Autodesk Fusion 360 part; units mm, degrees
note: some values were not read from the file. Set by a fixed rule: which face or edge a step refers to.
(part 12 of 12)
sketch "Sketch1 (2)" plane through (0, 0, 0) normal (0, 0, 1) x (1, 0, 0) in component "Component"
  spline S0 degree 5 poles (12.8573, -1.2306) (12.8574, -1.2306) (12.8577, -1.2307) (12.8582, -1.2307) (12.8589, -1.2308) (12.8601, -1.2308) (12.8614, -1.2309) (12.8628, -1.231) (12.8645, -1.2311) (12.8663, -1.2312) (12.8683, -1.2313) (12.8704, -1.2315) (12.8727, -1.2316) (12.8752, -1.2317) (12.8778, -1.2318) (12.8806, -1.2319) (12.8835, -1.232) (12.8866, -1.2321) (12.8898, -1.2321) (12.8931, -1.2322) (12.8966, -1.2323) (12.9003, -1.2323) (12.904, -1.2324) (12.9079, -1.2324) (12.912, -1.2324) (12.9161, -1.2324) (12.9204, -1.2324) (12.9248, -1.2324) (12.9294, -1.2323) (12.9341, -1.2323) (12.9389, -1.2322) (12.9438, -1.2321) (12.9488, -1.232) (12.954, -1.2318) (12.9592, -1.2317) (12.9646, -1.2315) (12.9701, -1.2313) (12.9757, -1.2311) (12.9814, -1.2309) (12.9873, -1.2306) (12.9932, -1.2303) (12.9992, -1.23) (13.0054, -1.2296) (13.0117, -1.2293) (13.018, -1.2289) (13.0245, -1.2285) (13.031, -1.228) (13.0377, -1.2276) (13.0444, -1.2271) (13.0513, -1.2265) (13.0583, -1.226) (13.0653, -1.2254) (13.0724, -1.2248) (13.0797, -1.2241) (13.087, -1.2234) (13.0944, -1.2227) (13.1019, -1.222) (13.1095, -1.2212) (13.1172, -1.2204) (13.125, -1.2196) (13.1329, -1.2187) (13.1408, -1.2178) (13.1488, -1.2169) (13.157, -1.2159) (13.1652, -1.2149) (13.1734, -1.2138) (13.1818, -1.2128) (13.1903, -1.2117) (13.1988, -1.2105) (13.2074, -1.2093) (13.2161, -1.2081) (13.2248, -1.2068) (13.2337, -1.2056) (13.2426, -1.2042) (13.2516, -1.2029) (13.2606, -1.2014) (13.2698, -1.2) (13.279, -1.1985) (13.2883, -1.197) (13.2976, -1.1954) (13.307, -1.1938) (13.3165, -1.1922) (13.3261, -1.1905) (13.3358, -1.1888) (13.3455, -1.187) (13.3552, -1.1852) (13.3651, -1.1834) (13.375, -1.1815) (13.385, -1.1796) (13.395, -1.1776) (13.4051, -1.1756) (13.4153, -1.1736) (13.4255, -1.1715) (13.4358, -1.1694) (13.4462, -1.1672) (13.4566, -1.165) (13.4671, -1.1627) (13.4776, -1.1604) (13.4882, -1.1581) (13.4989, -1.1557) (13.5096, -1.1533) (13.5204, -1.1508) (13.5312, -1.1483) (13.5421, -1.1457) (13.5531, -1.1431) (13.5641, -1.1404) (13.5752, -1.1377) (13.5863, -1.135) (13.5975, -1.1322) (13.6087, -1.1294) (13.62, -1.1265) (13.6313, -1.1236) (13.6427, -1.1206) (13.6542, -1.1176) (13.6657, -1.1146) (13.6772, -1.1115) (13.6888, -1.1083) (13.7005, -1.1051) (13.7122, -1.1019) (13.7239, -1.0986) (13.7357, -1.0953) (13.7476, -1.0919) (13.7595, -1.0885) (13.7714, -1.085) (13.7834, -1.0815) (13.7955, -1.0779) (13.8076, -1.0743) (13.8197, -1.0706) (13.8319, -1.0669) (13.8441, -1.0631) (13.8564, -1.0593) (13.8687, -1.0555) (13.8811, -1.0516) (13.8935, -1.0476) (13.9059, -1.0436) (13.9184, -1.0396) (13.931, -1.0355) (13.9435, -1.0314) (13.9562, -1.0272) (13.9688, -1.0229) (13.9815, -1.0186) (13.9943, -1.0143) (14.0071, -1.0099) (14.0199, -1.0055) (14.0328, -1.001) (14.0457, -0.9965) (14.0586, -0.9919) (14.0716, -0.9873) (14.0846, -0.9826) (14.0977, -0.9778) (14.1108, -0.9731) (14.1239, -0.9682) (14.1371, -0.9634) (14.1503, -0.9584) (14.1635, -0.9534) (14.1768, -0.9484) (14.1901, -0.9433) (14.2035, -0.9382) (14.2168, -0.933) (14.2303, -0.9278) (14.2437, -0.9225) (14.2572, -0.9172) (14.2707, -0.9118) (14.2843, -0.9064) (14.2979, -0.9009) (14.3115, -0.8954) (14.3251, -0.8898) (14.3388, -0.8842) (14.3525, -0.8785) (14.3663, -0.8727) (14.38, -0.8669) (14.3938, -0.8611) (14.4077, -0.8552) (14.4216, -0.8493) (14.4354, -0.8433) (14.4494, -0.8373) (14.4633, -0.8312) (14.4773, -0.825) (14.4913, -0.8188) (14.5054, -0.8126) (14.5194, -0.8063) (14.5335, -0.7999) (14.5476, -0.7935) (14.5618, -0.7871) (14.576, -0.7806) (14.5902, -0.774) (14.6044, -0.7674) (14.6186, -0.7608) (14.6329, -0.754) (14.6472, -0.7473) (14.6615, -0.7405) (14.6759, -0.7336) (14.6903, -0.7267) (14.7047, -0.7197) (14.7191, -0.7127) (14.7336, -0.7056) (14.748, -0.6985) (14.7625, -0.6913) (14.777, -0.6841) (14.7916, -0.6768) (14.8061, -0.6695) (14.8207, -0.6621) (14.8353, -0.6547) (14.8499, -0.6472) (14.8646, -0.6396) (14.8793, -0.632) (14.894, -0.6244) (14.9087, -0.6167) (14.9234, -0.609) (14.9381, -0.6011) (14.9529, -0.5933) (14.9677, -0.5854) (14.9825, -0.5774) (14.9973, -0.5694) (15.0122, -0.5614) (15.027, -0.5532) (15.0419, -0.5451) (15.0568, -0.5368) (15.0717, -0.5286) (15.0867, -0.5202) (15.1016, -0.5119) (15.1166, -0.5034) (15.1316, -0.495) (15.1466, -0.4864) (15.1616, -0.4778) (15.1766, -0.4692) (15.1916, -0.4605) (15.2067, -0.4518) (15.2218, -0.443) (15.2369, -0.4341) (15.252, -0.4252) (15.2671, -0.4162) (15.2822, -0.4072) (15.2974, -0.3982) (15.3125, -0.3891) (15.3277, -0.3799) (15.3429, -0.3707) (15.3581, -0.3614) (15.3733, -0.3521) (15.3885, -0.3427) (15.4038, -0.3333) (15.416, -0.3257) (15.4251, -0.32) (15.4312, -0.3162) (15.4343, -0.3143) knots 0 0 0 0 0 0 0.00416667 0.00833333 0.0125 0.01666667 0.02083333 0.025 0.02916667 0.03333333 0.0375 0.04166667 0.04583333 0.05 0.05416667 0.05833333 0.0625 0.06666667 0.07083333 0.075 0.07916667 0.08333333 0.0875 0.09166667 0.09583333 0.1 0.10416667 0.10833333 0.1125 0.11666667 0.12083333 0.125 0.12916667 0.13333333 0.1375 0.14166667 0.14583333 0.15 0.15416667 0.15833333 0.1625 0.16666667 0.17083333 0.175 0.17916667 0.18333333 0.1875 0.19166667 0.19583333 0.2 0.20416667 0.20833333 0.2125 0.21666667 0.22083333 0.225 0.22916667 0.23333333 0.2375 0.24166667 0.24583333 0.25 0.25416667 0.25833333 0.2625 0.26666667 0.27083333 0.275 0.27916667 0.28333333 0.2875 0.29166667 0.29583333 0.3 0.30416667 0.30833333 0.3125 0.31666667 0.32083333 0.325 0.32916667 0.33333333 0.3375 0.34166667 0.34583333 0.35 0.35416667 0.35833333 0.3625 0.36666667 0.37083333 0.375 0.37916667 0.38333333 0.3875 0.39166667 0.39583333 0.4 0.40416667 0.40833333 0.4125 0.41666667 0.42083333 0.425 0.42916667 0.43333333 0.4375 0.44166667 0.44583333 0.45 0.45416667 0.45833333 0.4625 0.46666667 0.47083333 0.475 0.47916667 0.48333333 0.4875 0.49166667 0.49583333 0.5 0.50416667 0.50833333 0.5125 0.51666667 0.52083333 0.525 0.52916667 0.53333333 0.5375 0.54166667 0.54583333 0.55 0.55416667 0.55833333 0.5625 0.56666667 0.57083333 0.575 0.57916667 0.58333333 0.5875 0.59166667 0.59583333 0.6 0.60416667 0.60833333 0.6125 0.61666667 0.62083333 0.625 0.62916667 0.63333333 0.6375 0.64166667 0.64583333 0.65 0.65416667 0.65833333 0.6625 0.66666667 0.67083333 0.675 0.67916667 0.68333333 0.6875 0.69166667 0.69583333 0.7 0.70416667 0.70833333 0.7125 0.71666667 0.72083333 0.725 0.72916667 0.73333333 0.7375 0.74166667 0.74583333 0.75 0.75416667 0.75833333 0.7625 0.76666667 0.77083333 0.775 0.77916667 0.78333333 0.7875 0.79166667 0.79583333 0.8 0.80416667 0.80833333 0.8125 0.81666667 0.82083333 0.825 0.82916667 0.83333333 0.8375 0.84166667 0.84583333 0.85 0.85416667 0.85833333 0.8625 0.86666667 0.87083333 0.875 0.87916667 0.88333333 0.8875 0.89166667 0.89583333 0.9 0.90416667 0.90833333 0.9125 0.91666667 0.92083333 0.925 0.92916667 0.93333333 0.9375 0.94166667 0.94583333 0.95 0.95416667 0.95833333 0.9625 0.96666667 0.97083333 0.975 0.97916667 0.98333333 0.9875 0.99166667 0.99583333 1 1 1 1 1 1
  spline S1 degree 5 poles (12.8573, 1.2306) (12.8574, 1.2306) (12.8577, 1.2307) (12.8582, 1.2307) (12.8589, 1.2308) (12.8601, 1.2308) (12.8614, 1.2309) (12.8628, 1.231) (12.8645, 1.2311) (12.8663, 1.2312) (12.8683, 1.2313) (12.8704, 1.2315) (12.8727, 1.2316) (12.8752, 1.2317) (12.8778, 1.2318) (12.8806, 1.2319) (12.8835, 1.232) (12.8866, 1.2321) (12.8898, 1.2321) (12.8931, 1.2322) (12.8966, 1.2323) (12.9003, 1.2323) (12.904, 1.2324) (12.9079, 1.2324) (12.912, 1.2324) (12.9161, 1.2324) (12.9204, 1.2324) (12.9248, 1.2324) (12.9294, 1.2323) (12.9341, 1.2323) (12.9389, 1.2322) (12.9438, 1.2321) (12.9488, 1.232) (12.954, 1.2318) (12.9592, 1.2317) (12.9646, 1.2315) (12.9701, 1.2313) (12.9757, 1.2311) (12.9814, 1.2309) (12.9873, 1.2306) (12.9932, 1.2303) (12.9992, 1.23) (13.0054, 1.2296) (13.0117, 1.2293) (13.018, 1.2289) (13.0245, 1.2285) (13.031, 1.228) (13.0377, 1.2276) (13.0444, 1.2271) (13.0513, 1.2265) (13.0583, 1.226) (13.0653, 1.2254) (13.0724, 1.2248) (13.0797, 1.2241) (13.087, 1.2234) (13.0944, 1.2227) (13.1019, 1.222) (13.1095, 1.2212) (13.1172, 1.2204) (13.125, 1.2196) (13.1329, 1.2187) (13.1408, 1.2178) (13.1488, 1.2169) (13.157, 1.2159) (13.1652, 1.2149) (13.1734, 1.2138) (13.1818, 1.2128) (13.1903, 1.2117) (13.1988, 1.2105) (13.2074, 1.2093) (13.2161, 1.2081) (13.2248, 1.2068) (13.2337, 1.2056) (13.2426, 1.2042) (13.2516, 1.2029) (13.2606, 1.2014) (13.2698, 1.2) (13.279, 1.1985) (13.2883, 1.197) (13.2976, 1.1954) (13.307, 1.1938) (13.3165, 1.1922) (13.3261, 1.1905) (13.3358, 1.1888) (13.3455, 1.187) (13.3552, 1.1852) (13.3651, 1.1834) (13.375, 1.1815) (13.385, 1.1796) (13.395, 1.1776) (13.4051, 1.1756) (13.4153, 1.1736) (13.4255, 1.1715) (13.4358, 1.1694) (13.4462, 1.1672) (13.4566, 1.165) (13.4671, 1.1627) (13.4776, 1.1604) (13.4882, 1.1581) (13.4989, 1.1557) (13.5096, 1.1533) (13.5204, 1.1508) (13.5312, 1.1483) (13.5421, 1.1457) (13.5531, 1.1431) (13.5641, 1.1404) (13.5752, 1.1377) (13.5863, 1.135) (13.5975, 1.1322) (13.6087, 1.1294) (13.62, 1.1265) (13.6313, 1.1236) (13.6427, 1.1206) (13.6542, 1.1176) (13.6657, 1.1146) (13.6772, 1.1115) (13.6888, 1.1083) (13.7005, 1.1051) (13.7122, 1.1019) (13.7239, 1.0986) (13.7357, 1.0953) (13.7476, 1.0919) (13.7595, 1.0885) (13.7714, 1.085) (13.7834, 1.0815) (13.7955, 1.0779) (13.8076, 1.0743) (13.8197, 1.0706) (13.8319, 1.0669) (13.8441, 1.0631) (13.8564, 1.0593) (13.8687, 1.0555) (13.8811, 1.0516) (13.8935, 1.0476) (13.9059, 1.0436) (13.9184, 1.0396) (13.931, 1.0355) (13.9435, 1.0314) (13.9562, 1.0272) (13.9688, 1.0229) (13.9815, 1.0186) (13.9943, 1.0143) (14.0071, 1.0099) (14.0199, 1.0055) (14.0328, 1.001) (14.0457, 0.9965) (14.0586, 0.9919) (14.0716, 0.9873) (14.0846, 0.9826) (14.0977, 0.9778) (14.1108, 0.9731) (14.1239, 0.9682) (14.1371, 0.9634) (14.1503, 0.9584) (14.1635, 0.9534) (14.1768, 0.9484) (14.1901, 0.9433) (14.2035, 0.9382) (14.2168, 0.933) (14.2303, 0.9278) (14.2437, 0.9225) (14.2572, 0.9172) (14.2707, 0.9118) (14.2843, 0.9064) (14.2979, 0.9009) (14.3115, 0.8954) (14.3251, 0.8898) (14.3388, 0.8842) (14.3525, 0.8785) (14.3663, 0.8727) (14.38, 0.8669) (14.3938, 0.8611) (14.4077, 0.8552) (14.4216, 0.8493) (14.4354, 0.8433) (14.4494, 0.8373) (14.4633, 0.8312) (14.4773, 0.825) (14.4913, 0.8188) (14.5054, 0.8126) (14.5194, 0.8063) (14.5335, 0.7999) (14.5476, 0.7935) (14.5618, 0.7871) (14.576, 0.7806) (14.5902, 0.774) (14.6044, 0.7674) (14.6186, 0.7608) (14.6329, 0.754) (14.6472, 0.7473) (14.6615, 0.7405) (14.6759, 0.7336) (14.6903, 0.7267) (14.7047, 0.7197) (14.7191, 0.7127) (14.7336, 0.7056) (14.748, 0.6985) (14.7625, 0.6913) (14.777, 0.6841) (14.7916, 0.6768) (14.8061, 0.6695) (14.8207, 0.6621) (14.8353, 0.6547) (14.8499, 0.6472) (14.8646, 0.6396) (14.8793, 0.632) (14.894, 0.6244) (14.9087, 0.6167) (14.9234, 0.609) (14.9381, 0.6011) (14.9529, 0.5933) (14.9677, 0.5854) (14.9825, 0.5774) (14.9973, 0.5694) (15.0122, 0.5614) (15.027, 0.5532) (15.0419, 0.5451) (15.0568, 0.5368) (15.0717, 0.5286) (15.0867, 0.5202) (15.1016, 0.5119) (15.1166, 0.5034) (15.1316, 0.495) (15.1466, 0.4864) (15.1616, 0.4778) (15.1766, 0.4692) (15.1916, 0.4605) (15.2067, 0.4518) (15.2218, 0.443) (15.2369, 0.4341) (15.252, 0.4252) (15.2671, 0.4162) (15.2822, 0.4072) (15.2974, 0.3982) (15.3125, 0.3891) (15.3277, 0.3799) (15.3429, 0.3707) (15.3581, 0.3614) (15.3733, 0.3521) (15.3885, 0.3427) (15.4038, 0.3333) (15.416, 0.3257) (15.4251, 0.32) (15.4312, 0.3162) (15.4343, 0.3143) knots 0 0 0 0 0 0 0.00416667 0.00833333 0.0125 0.01666667 0.02083333 0.025 0.02916667 0.03333333 0.0375 0.04166667 0.04583333 0.05 0.05416667 0.05833333 0.0625 0.06666667 0.07083333 0.075 0.07916667 0.08333333 0.0875 0.09166667 0.09583333 0.1 0.10416667 0.10833333 0.1125 0.11666667 0.12083333 0.125 0.12916667 0.13333333 0.1375 0.14166667 0.14583333 0.15 0.15416667 0.15833333 0.1625 0.16666667 0.17083333 0.175 0.17916667 0.18333333 0.1875 0.19166667 0.19583333 0.2 0.20416667 0.20833333 0.2125 0.21666667 0.22083333 0.225 0.22916667 0.23333333 0.2375 0.24166667 0.24583333 0.25 0.25416667 0.25833333 0.2625 0.26666667 0.27083333 0.275 0.27916667 0.28333333 0.2875 0.29166667 0.29583333 0.3 0.30416667 0.30833333 0.3125 0.31666667 0.32083333 0.325 0.32916667 0.33333333 0.3375 0.34166667 0.34583333 0.35 0.35416667 0.35833333 0.3625 0.36666667 0.37083333 0.375 0.37916667 0.38333333 0.3875 0.39166667 0.39583333 0.4 0.40416667 0.40833333 0.4125 0.41666667 0.42083333 0.425 0.42916667 0.43333333 0.4375 0.44166667 0.44583333 0.45 0.45416667 0.45833333 0.4625 0.46666667 0.47083333 0.475 0.47916667 0.48333333 0.4875 0.49166667 0.49583333 0.5 0.50416667 0.50833333 0.5125 0.51666667 0.52083333 0.525 0.52916667 0.53333333 0.5375 0.54166667 0.54583333 0.55 0.55416667 0.55833333 0.5625 0.56666667 0.57083333 0.575 0.57916667 0.58333333 0.5875 0.59166667 0.59583333 0.6 0.60416667 0.60833333 0.6125 0.61666667 0.62083333 0.625 0.62916667 0.63333333 0.6375 0.64166667 0.64583333 0.65 0.65416667 0.65833333 0.6625 0.66666667 0.67083333 0.675 0.67916667 0.68333333 0.6875 0.69166667 0.69583333 0.7 0.70416667 0.70833333 0.7125 0.71666667 0.72083333 0.725 0.72916667 0.73333333 0.7375 0.74166667 0.74583333 0.75 0.75416667 0.75833333 0.7625 0.76666667 0.77083333 0.775 0.77916667 0.78333333 0.7875 0.79166667 0.79583333 0.8 0.80416667 0.80833333 0.8125 0.81666667 0.82083333 0.825 0.82916667 0.83333333 0.8375 0.84166667 0.84583333 0.85 0.85416667 0.85833333 0.8625 0.86666667 0.87083333 0.875 0.87916667 0.88333333 0.8875 0.89166667 0.89583333 0.9 0.90416667 0.90833333 0.9125 0.91666667 0.92083333 0.925 0.92916667 0.93333333 0.9375 0.94166667 0.94583333 0.95 0.95416667 0.95833333 0.9625 0.96666667 0.97083333 0.975 0.97916667 0.98333333 0.9875 0.99166667 0.99583333 1 1 1 1 1 1
  spline S2 degree 5 poles (12.8561, -1.2305) (12.8562, -1.2305) (12.8563, -1.2305) (12.8564, -1.2306) (12.8566, -1.2306) (12.8568, -1.2306) (12.857, -1.2306) (12.8571, -1.2306) (12.8572, -1.2306) (12.8573, -1.2306) knots 0 0 0 0 0 0 0.2 0.4 0.6 0.8 1 1 1 1 1 1
  spline S3 degree 5 poles (12.8561, 1.2305) (12.8562, 1.2305) (12.8563, 1.2305) (12.8564, 1.2306) (12.8566, 1.2306) (12.8568, 1.2306) (12.857, 1.2306) (12.8571, 1.2306) (12.8572, 1.2306) (12.8573, 1.2306) knots 0 0 0 0 0 0 0.2 0.4 0.6 0.8 1 1 1 1 1 1
  line L0 (0, 0) -> (12.8561, -1.2305)
  line L1 (0, 0) -> (12.8561, 1.2305)
  arc A0 (15.4343, -0.3143) -> (15.4343, 0.3143) centre (0, 0) ccw
  point P0 (12.8607, -1.2309)
  point P1 (12.8665, -1.2312)
  point P2 (12.8745, -1.2316)
  point P3 (12.8849, -1.232)
  point P4 (12.8976, -1.2323)
  point P5 (12.9126, -1.2324)
  point P6 (12.9299, -1.2323)
  point P7 (12.9495, -1.232)
  point P8 (12.9714, -1.2313)
  point P9 (12.9956, -1.2302)
  point P10 (13.0221, -1.2286)
  point P11 (13.0508, -1.2266)
  point P12 (13.0819, -1.2239)
  point P13 (13.1151, -1.2206)
  point P14 (13.1507, -1.2166)
  point P15 (13.1884, -1.2119)
  point P16 (13.2284, -1.2063)
  point P17 (13.2706, -1.1999)
  point P18 (13.3149, -1.1925)
  point P19 (13.3615, -1.1841)
  point P20 (13.4102, -1.1746)
  point P21 (13.461, -1.164)
  point P22 (13.5139, -1.1523)
  point P23 (13.5689, -1.1393)
  point P24 (13.6259, -1.125)
  point P25 (13.685, -1.1093)
  point P26 (13.7461, -1.0923)
  point P27 (13.8092, -1.0738)
  point P28 (13.8742, -1.0538)
  point P29 (13.9412, -1.0321)
  point P30 (14.01, -1.0089)
  point P31 (14.0807, -0.984)
  point P32 (14.1532, -0.9573)
  point P33 (14.2275, -0.9289)
  point P34 (14.3036, -0.8986)
  point P35 (14.3814, -0.8664)
  point P36 (14.4609, -0.8322)
  point P37 (14.542, -0.7961)
  point P38 (14.6247, -0.7579)
  point P39 (14.709, -0.7176)
  point P40 (14.7948, -0.6752)
  point P41 (14.8821, -0.6306)
  point P42 (14.9708, -0.5837)
  point P43 (15.0609, -0.5346)
  point P44 (15.1523, -0.4831)
  point P45 (15.2451, -0.4293)
  point P46 (15.3391, -0.373)
  point P47 (12.8607, 1.2309)
  point P48 (12.8665, 1.2312)
  point P49 (12.8745, 1.2316)
  point P50 (12.8849, 1.232)
  point P51 (12.8976, 1.2323)
  point P52 (12.9126, 1.2324)
  point P53 (12.9299, 1.2323)
  point P54 (12.9495, 1.232)
  point P55 (12.9714, 1.2313)
  point P56 (12.9956, 1.2302)
  point P57 (13.0221, 1.2286)
  point P58 (13.0508, 1.2266)
  point P59 (13.0819, 1.2239)
  point P60 (13.1151, 1.2206)
  point P61 (13.1507, 1.2166)
  point P62 (13.1884, 1.2119)
  point P63 (13.2284, 1.2063)
  point P64 (13.2706, 1.1999)
  point P65 (13.3149, 1.1925)
  point P66 (13.3615, 1.1841)
  point P67 (13.4102, 1.1746)
  point P68 (13.461, 1.164)
  point P69 (13.5139, 1.1523)
  point P70 (13.5689, 1.1393)
  point P71 (13.6259, 1.125)
  point P72 (13.685, 1.1093)
  point P73 (13.7461, 1.0923)
  point P74 (13.8092, 1.0738)
  point P75 (13.8742, 1.0538)
  point P76 (13.9412, 1.0321)
  point P77 (14.01, 1.0089)
  point P78 (14.0807, 0.984)
  point P79 (14.1532, 0.9573)
  point P80 (14.2275, 0.9289)
  point P81 (14.3036, 0.8986)
  point P82 (14.3814, 0.8664)
  point P83 (14.4609, 0.8322)
  point P84 (14.542, 0.7961)
  point P85 (14.6247, 0.7579)
  point P86 (14.709, 0.7176)
  point P87 (14.7948, 0.6752)
  point P88 (14.8821, 0.6306)
  point P89 (14.9708, 0.5837)
  point P90 (15.0609, 0.5346)
  point P91 (15.1523, 0.4831)
  point P92 (15.2451, 0.4293)
  point P93 (15.3391, 0.373)
sketch "Sketch2" plane through (0, 0, 0) normal (0, 0, 1) x (1, 0, 0) in component "Component"
  circle A0 centre (0, 0) radius 12.7656
extrude "Extrude1" add sketch "Sketch2" along normal blind 5 makes body 1 in component "Component"
extrude "Extrude2" add sketch "Sketch1 (2)" along normal blind 5 separate body makes body 2 in component "Component"
pattern_circular "C-Pattern1" count 24 over 360 about axis through (0, 0, 1.75) along (0, 0, 1) of "Extrude2" makes body 3 at (4.0336, 1.5055, 1.6667) makes body 4 at (3.9167, 1.7876, 1.6667) makes body 5 at (3.3206, 2.7404, 1.6667) makes body 6 at (2.4981, 3.5065, 3.3333) makes body 7 at (0.713, 4.2459, 1.6667) makes body 8 at (0.4102, 4.2858, 1.6667) makes body 9 at (-0.713, 4.2459, 1.6667) makes body 10 at (-1.7876, 3.9167, 1.6667) makes body 11 at (-2.7404, 3.3206, 1.6667) makes body 12 at (-3.5065, 2.4981, 1.6667) makes body 13 at (-4.0336, 1.5055, 1.6667) makes body 14 at (-4.2858, 0.4102, 1.6667) makes body 15 at (-4.2459, -0.713, 1.6667) makes body 16 at (-3.9167, -1.7876, 1.6667) makes body 17 at (-3.3206, -2.7404, 1.6667) makes body 18 at (-1.7876, -3.9167, 1.6667) makes body 19 at (-0.713, -4.2459, 1.6667) makes body 20 at (-0.4102, -4.2858, 1.6667) makes body 21 at (0.713, -4.2459, 1.6667) makes body 22 at (1.7876, -3.9167, 1.6667) makes body 23 at (2.7404, -3.3206, 1.6667) makes body 24 at (3.9167, -1.7876, 1.6667) makes body 25 at (4.0336, -1.5055, 1.6667) in component "Component"
combine "Combine1" operation add target body 1 tool bodies 2 3 4 5 6 7 8 9 10 11 12 13 14 15 16 17 18 19 20 21 22 23 24 25 in component "Component"
sketch "Sketch3" plane through (0, 0, 0) normal (0, 0, 1) x (1, 0, 0) in component "Component"
  line L0 (0, 0) -> (52.5498, 0) construction
  line L1 (52.5498, 0) -> (52.5498, 3) construction
  line L2 (52.5498, 3) -> (0, 3) construction
  line L3 (0, 3) -> (0, 0) construction
  constraint perpendicular L0 L1
  constraint parallel L0 L2
  constraint parallel L1 L3
extrude "Extrude3" cut sketch "Sketch1" against normal blind 6 contours A24 | A25 | A26 | A27 | A28 bodies 1 in component "Component"
extrude "Extrude4" cut sketch "Sketch1" against normal blind 4 contours A29 bodies 1 in component "Component"
component "Component" placed x (1, 0, 0) y (0, 1, 0) z (0, 0, 1) at (0, 0, 0)
component "Component" placed x (1, 0, 0) y (0, 1, 0) z (0, 0, 1) at (0, 34, 0)

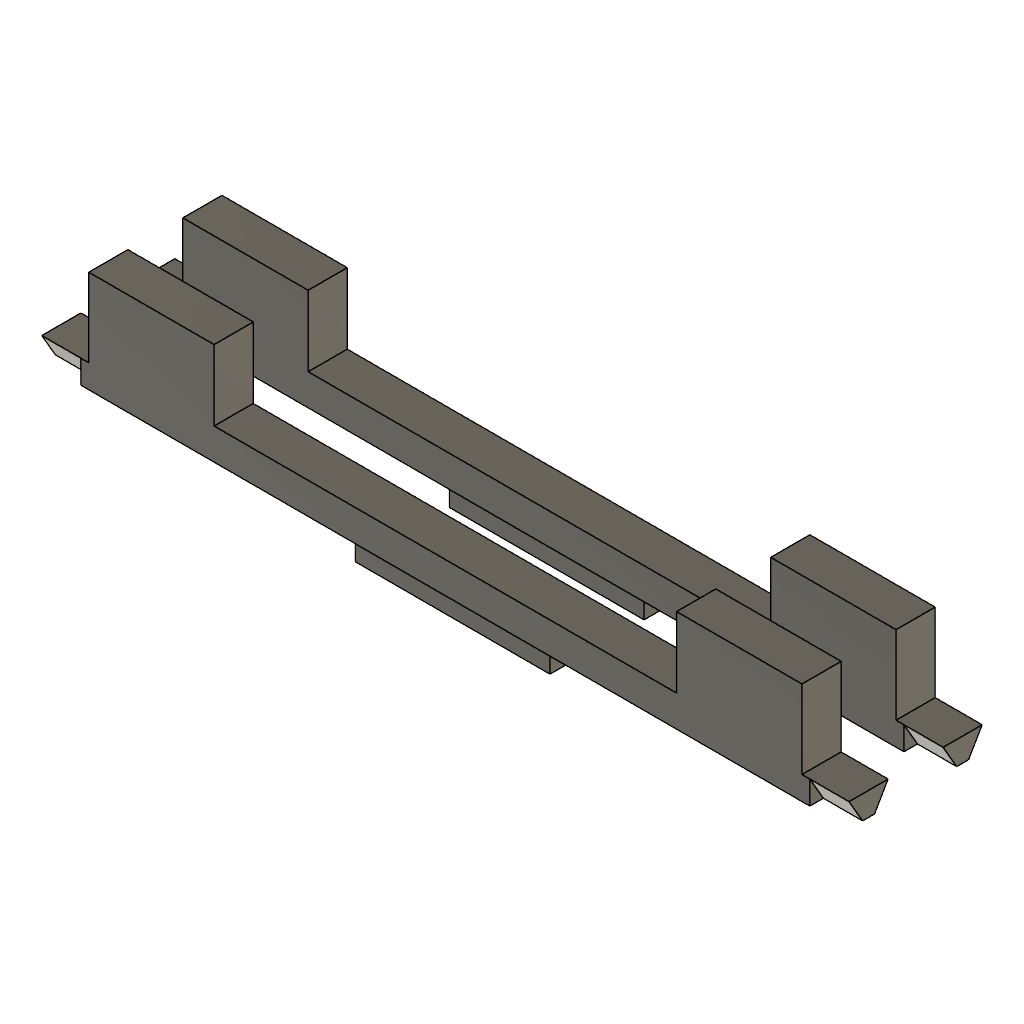
design "card-shuffler-inner-walls"
part number: 2026-07-29-15-03-19-549
part number: 2026-08-01-04-48-56-794
Autodesk Fusion 360 part; units mm, degrees
sketch "Sketch2" plane through (0, 0, 0) normal (0, 0, 1) x (1, 0, 0)
  line L0 (0, 0) -> (6, 0)
  line L1 (6, 0) -> (6, 5)
  line L2 (6, 5) -> (0, 5)
  line L3 (0, 5) -> (0, 0)
  line L4 (6, 5) -> (22, 5)
  line L5 (22, 5) -> (22, 0)
  line L6 (22, 0) -> (6, 0)
  line L7 (6, 0) -> (6, 5)
  line L8 (22, 5) -> (43, 5)
  line L9 (43, 5) -> (43, 0)
  line L10 (43, 0) -> (22, 0)
  line L11 (22, 0) -> (22, 5)
  line L12 (43, 5) -> (60, 5)
  line L13 (60, 5) -> (60, 0)
  line L14 (60, 0) -> (43, 0)
  line L15 (43, 0) -> (43, 5)
  line L16 (60, 5) -> (81, 5)
  line L17 (81, 5) -> (81, 0)
  line L18 (81, 0) -> (60, 0)
  line L19 (60, 0) -> (60, 5)
  line L20 (81, 5) -> (97, 5)
  line L21 (97, 5) -> (97, 0)
  line L22 (97, 0) -> (81, 0)
  line L23 (81, 0) -> (81, 5)
  line L24 (97, 5) -> (103, 5)
  line L25 (103, 5) -> (103, 0)
  line L26 (103, 0) -> (97, 0)
  line L27 (97, 0) -> (97, 5)
  dimension "d22" = 6
  dimension "d23" = 16
  dimension "d24" = 21
  dimension "d25" = 17
  dimension "d26" = 21
  dimension "d27" = 16
  dimension "d28" = 6
  constraint horizontal L0
  constraint vertical L1
  constraint horizontal L2
  constraint vertical L3
  constraint coincident L0.start L3.end
  constraint horizontal L4
  constraint vertical L5
  constraint horizontal L6
  constraint vertical L7
  constraint horizontal L8
  constraint vertical L9
  constraint horizontal L10
  constraint vertical L11
  constraint horizontal L12
  constraint vertical L13
  constraint horizontal L14
  constraint vertical L15
  constraint horizontal L16
  constraint vertical L17
  constraint horizontal L18
  constraint vertical L19
  constraint horizontal L20
  constraint vertical L21
  constraint horizontal L22
  constraint vertical L23
  constraint horizontal L24
  constraint vertical L25
  constraint horizontal L26
  constraint vertical L27
  measures "d22" distance of L3 L7
  measures "d23" distance of L5 L7
  measures "d24" distance of L5 L15
  measures "d25" distance of L13 L15
  measures "d26" distance of L17 L19
  measures "d27" distance of L21 L23
  measures "d28" distance of L21 L25
extrude "Extrude3" add sketch "Sketch2" against normal blind 3 makes body 1
extrude "Extrude4" add sketch "Sketch2" along normal blind 10 contours L1 L4 L5 L6 L7 L11 | L17 L20 L21 L22 L23 L27 bodies 1
extrude "Extrude10" add 1 faces at (41.6667, 3.3333, 0) along direction (0, 0, 1) blind 1 on bodies 1 bodies 1
sketch "Sketch3" plane through (103, 0, 0) normal (1, 0, 0) x (0, 1, 0)
  line L0 (5, 0) -> (0, 0)
  line L1 (0, 0) -> (0, -3)
  line L2 (0, -3) -> (5, -3)
  line L3 (5, -3) -> (5, 0)
  line L4 (0, 0) -> (2.5, -4.3301)
  line L5 (2.5, -4.3301) -> (5, 0)
  line L6 (5, 0) -> (0, 0)
  point P0 (2.5, -1.4434)
  constraint coincident L0.end L1.start
  constraint coincident L0.start L3.end
extrude "Extrude5" cut sketch "Sketch3" against normal blind 5 contours L2 L3 L5 | L1 L2 L4 bodies 1
sketch "Sketch4" plane through (0, 0, 0) normal (-1, 0, 0) x (0, -1, 0)
  line L0 (0, 0) -> (-5, 0)
  line L1 (-5, 0) -> (-5, -3)
  line L2 (-5, -3) -> (0, -3)
  line L3 (0, -3) -> (0, 0)
  line L4 (-5, 0) -> (-2.5, -4.3301)
  line L5 (-2.5, -4.3301) -> (0, 0)
  line L6 (0, 0) -> (-5, 0)
  point P0 (-2.5, -1.4434)
  constraint coincident L0.start L3.end
  constraint coincident L0.end L1.start
extrude "Extrude8" cut sketch "Sketch4" against normal blind 5 contours L2 L3 L5 | L1 L2 L4 bodies 1
sketch "Sketch5" plane through (0, 0, -3) normal (0, 0, -1) x (1, 0, 0)
  line L0 (0, -3.2679) -> (5, -3.2679)
  line L1 (5, -3.2679) -> (5, -5)
  line L2 (5, -5) -> (98, -5)
  line L3 (98, -5) -> (98, -3.2679)
  line L4 (98, -3.2679) -> (103, -3.2679)
  line L5 (103, -3.2679) -> (103, -1.7321)
  line L6 (103, -1.7321) -> (98, -1.7321)
  line L7 (98, -1.7321) -> (98, 0)
  line L8 (98, 0) -> (5, 0)
  line L9 (5, 0) -> (5, -1.7321)
  line L10 (5, -1.7321) -> (0, -1.7321)
  line L11 (0, -1.7321) -> (0, -3.2679)
  line L12 (5, 0) -> (98, 0)
  line L13 (98, 0) -> (98, -5)
  line L14 (98, -5) -> (5, -5)
  line L15 (5, -5) -> (5, 0)
  line L16 (63.85, -1) -> (39, -1)
  line L17 (39, -1) -> (39, -3.85)
  line L18 (39, -3.85) -> (63.85, -3.85)
  line L19 (63.85, -3.85) -> (63.85, -1)
  line L20 (63.85, -1) -> (39, -3.85) construction
  line L21 (39, -1) -> (63.85, -3.85) construction
  point P0 (51.425, -2.425)
  dimension "d44" = 24.85
  dimension "d45" = 2.85
  constraint horizontal L12
  constraint vertical L13
  constraint horizontal L14
  constraint vertical L15
  constraint coincident L2.end L3.start
  constraint coincident L8.end L9.start
  constraint horizontal L16
  constraint perpendicular L16 L17
  constraint parallel L16 L18
  constraint parallel L17 L19
  constraint coincident L20 P0
  constraint coincident L21 P0
  measures "d44" distance of L17.end L18.end
  measures "d45" distance of L16.end L17.end
extrude "Extrude9" add sketch "Sketch5" along normal blind 3 contours L16 L17 L18 L19 bodies 1
copy_body "Body->Comp3" bodies 1 removing the originals makes body 2 in component "Component"
component "Component" placed x (1, 0, 0) y (0, 1, 0) z (0, 0, 1) at (0, 0, 0)
component "Component" placed x (1, 0, 0) y (0, 1, 0) z (0, 0, 1) at (0, 12, 0)
